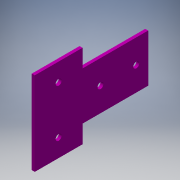
# Autodesk Inventor part: L Plate
Saved by Autodesk Inventor 2017 (Build 210142000, 142)
## iProperties
Created: 2017-01-21
Part Number: L Plate
Material: Aluminum 6061
Document SubType Name: Modeling
Designer: Ben
Density: 2.7 g/cm^3
Appearance: Magenta
Mass: 8.55474 g
Surface Area: 43.7504 cm^2
Volume: 3.16842 cm^3
Author: Ben
Autodesk Inventor part; units mm, degrees
ref_plane "YZ Plane" through (0, 0, 0) normal (1, 0, 0) x (0, 1, 0)
ref_plane "XZ Plane" through (0, 0, 0) normal (0, 1, 0) x (-1, 0, 0)
ref_plane "XY Plane" through (0, 0, 0) normal (0, 0, 1) x (1, 0, 0)
sketch "Sketch1" plane through (0, 0, 0) normal (1, 0, 0) x (0, 1, 0)
  line L0 (0, 0) -> (0, -41.275) construction
  circle A0 centre (0, -22.225) radius 1.5875
  circle A1 centre (0, -41.275) radius 1.5875
  line L1 (22.225, 12.7) -> (22.225, -12.7)
  line L2 (22.225, -12.7) -> (12.7, -12.7)
  line L3 (12.7, -12.7) -> (12.7, -47.625)
  line L4 (12.7, -47.625) -> (-12.7, -47.625)
  line L5 (-22.225, 12.7) -> (22.225, 12.7)
  line L6 (0, -41.275) -> (0, -47.625) construction
  line L7 (12.7, 0) -> (-12.7, 0) construction
  circle A2 centre (12.7, 0) radius 1.5875
  circle A3 centre (-12.7, 0) radius 1.5875
  line L8 (-22.225, 12.7) -> (-22.225, -12.7)
  line L9 (-22.225, -12.7) -> (-12.7, -12.7)
  line L10 (-12.7, -12.7) -> (-12.7, -47.625)
  dimension "d2" = 22.225
  dimension "d3" = 19.05
  dimension "d4" = 25.4
  dimension "d5" = 6.35
  dimension "d9" = 3.175
  dimension "d10" = 25.4
  dimension "d11" = 9.525
  dimension "d12" = 12.7
  constraints: 22 end point, 5 perpendicular, 4 centre point, 4 coincident, 4 vertical, 3 equal radius, 2 equal length, 2 horizontal, 2 midpoint, 1 collinear, 1 point on line
  measures "d2" distance of A0.centre point (0, 0)
  measures "d3" distance of A0.centre L0.end
  measures "d4" distance of L3.end L4.end
  measures "d5" distance from line of L0.end L4
  measures "d9" diameter of A2
  measures "d10" distance of L7.start L7.end
  measures "d11" distance from line of L7.start L1
  measures "d12" distance between parallel lines of L2 L7
extrude "Extrusion1" add sketch "Sketch1" along normal blind 1.5875
body "Solid1"
